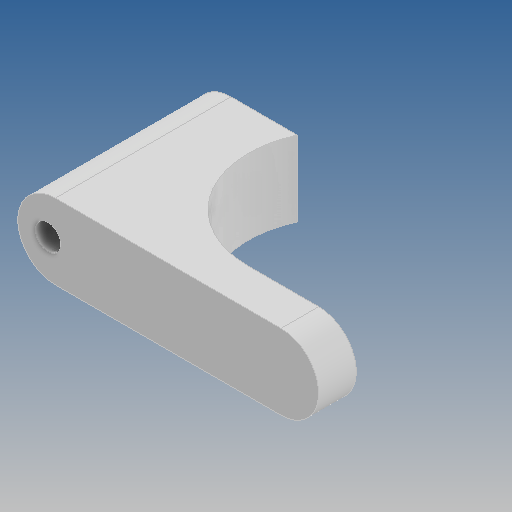
# Autodesk Inventor part: 0008-30-009
Saved by Autodesk Inventor 2020 (Build 240168000, 168)
## iProperties
Created: 2021-05-24
Part Number: 0008-30-009
Material: Generic
Document SubType Name: Modeling
Designer: Iulian Bors
Density: 1 g/cm^3
Appearance: Default
Author: Iulian Bors
Subject: 009
Autodesk Inventor part; units mm, degrees
ref_plane "YZ Plane" through (0, 0, 0) normal (1, 0, 0) x (0, 1, 0)
ref_plane "XZ Plane" through (0, 0, 0) normal (0, 1, 0) x (-1, 0, 0)
ref_plane "XY Plane" through (0, 0, 0) normal (0, 0, 1) x (1, 0, 0)
sketch "Sketch1" plane through (0, 0, 0) normal (0, 0, 1) x (1, 0, 0)
  line L0 (-30, 7.5) -> (30, 7.5)
  line L1 (30, 7.5) -> (30, -7.5)
  line L2 (30, -7.5) -> (-30, -7.5)
  line L3 (-30, -7.5) -> (-30, 7.5)
  circle A0 centre (-24, 0) radius 2.5
  point P0 (0, 0)
  point P1 (0, 7.5)
  point P2 (-30, 0)
  dimension "d0" = 5
  dimension "d1" = 6
  dimension "d2" = 15
  dimension "d3" = 60
  constraints: 8 end point, 2 horizontal alignment, 2 midpoint, 2 parallel, 1 centre point, 1 horizontal, 1 perpendicular, 1 vertical alignment
  measures "d0" diameter of A0
  measures "d1" distance from line of A0.centre L3
  measures "d2" distance of L2.end L0.start
  measures "d3" distance of L0.start L0.end
extrude "Extrusion1" add sketch "Sketch1" along normal blind 35
sketch "Sketch2" plane through (-30, -7.5, 0) normal (0, -1, 0) x (1, 0, 0)
  circle A0 centre (38.5, 8) radius 17.9938 projected
  arc A1 (38.5, 27.5) -> (56.2834, 0) centre (38.5, 8) ccw
  line L0 (38.5, 27.5) -> (60, 27.5)
  line L1 (60, 0) -> (60, 35) projected
  line L2 (0, 0) -> (60, 0) projected
  point P0 (30, 0)
  point P1 (20.7166, 0)
  dimension "d6" = 39
  constraints: 2 end point, 2 point on circle, 2 point on line, 1 centre point, 1 coincident, 1 perpendicular, 1 tangent
  measures "d6" diameter of A1
extrude "Extrusion2" cut sketch "Sketch2" against normal through all contours A0 L2 | A0 L2 A1 L0 L1 picked at (33.6467, 10.9183)
fillet "Fillet1" radius 7.5 4 edges at (-30, 7.5, 17.5) (-30, -7.5, 17.5) (30, -7.5, 31.25) (30, 7.5, 31.25)
body "Solid1"
